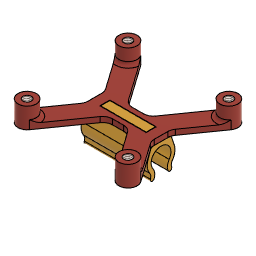
PixRacer Mount v3 (Autodesk Fusion 360 design; units mm, degrees)
Autodesk Fusion 360 part; units mm, degrees
note: some values were not read from the file. Chosen so that the rebuilt part matches the saved one: which face or edge a step refers to; which pieces of a blend or face edit are solid. Set by a fixed rule: which sketch regions a step uses.
sketch "Sketch1" plane through (0, 0, 0) normal (0, 0, 1) x (1, 0, 0)
  circle A0 centre (15.25, 15.25) radius 2.7625
  line L0 (0, 0) -> (0, 23.0197) construction
  line L1 (10, 3) -> (-10, 3)
  line L2 (-10, 3) -> (-10, -3)
  line L3 (-10, -3) -> (10, -3)
  line L4 (10, -3) -> (10, 3)
  line L5 (10, 3) -> (-10, -3) construction
  line L6 (-10, 3) -> (10, -3) construction
  line L7 (10, 3) -> (17.5084, 13.6591)
  line L8 (12.9916, 16.8409) -> (3.2419, 3)
  line L9 (0, 0) -> (10, 0)
  line L10 (10, -3) -> (17.5084, -13.6591)
  circle A1 centre (15.25, -15.25) radius 2.7625
  line L11 (12.9916, -16.8409) -> (3.2419, -3)
  line L12 (-10, 3) -> (-17.5084, 13.6591)
  circle A2 centre (-15.25, 15.25) radius 2.7625
  line L13 (-12.9916, 16.8409) -> (-3.2419, 3)
  line L14 (-10, -3) -> (-17.5084, -13.6591)
  line L15 (-12.9916, -16.8409) -> (-3.2419, -3)
  circle A3 centre (-15.25, -15.25) radius 2.7625
  line L16 (7, 1.5) -> (-7, 1.5)
  line L17 (-7, 1.5) -> (-7, -1.5)
  line L18 (-7, -1.5) -> (7, -1.5)
  line L19 (7, -1.5) -> (7, 1.5)
  line L20 (7, 1.5) -> (-7, -1.5) construction
  line L21 (-7, 1.5) -> (7, -1.5) construction
  dimension "d3" = 5.525
  dimension "d4" = 15.25
  dimension "d5" = 15.25
  dimension "d6" = 20
  dimension "d7" = 6
  dimension "d32" = 3
  dimension "d33" = 3
  constraint coincident L0.start L9.start
  constraint vertical L0
  constraint horizontal L1
  constraint perpendicular L1 L2
  constraint parallel L1 L3
  constraint parallel L2 L4
  constraint coincident L5 L0.start
  constraint coincident L6 L0.start
  constraint coincident A0 L7.end
  constraint tangent A0 L7
  constraint coincident A0 L8.start
  constraint coincident L1 L8.end
  constraint parallel L7 L8
  constraint tangent A0 L8
  constraint midpoint L4 L9.end
  constraint symmetric A0 L9 A1
  constraint symmetric L1.start L9 L3.end
  constraint symmetric L7.end L9 L10.end
  constraint symmetric L8.start L9 L11.start
  constraint symmetric L8.end L9 L11.end
  constraint symmetric A0 L0 A2
  constraint symmetric L0 L1.start L1.end
  constraint symmetric L0 L7.end L12.end
  constraint symmetric L0 L8.start L13.start
  constraint symmetric L0 L8.end L13.end
  constraint symmetric L0 L3.end L2.end
  constraint symmetric L0 L10.end L14.end
  constraint symmetric L0 A1 A3
  constraint symmetric L0 L11.start L15.start
  constraint symmetric L0 L11.end L15.end
  constraint horizontal L16
  constraint perpendicular L16 L17
  constraint parallel L16 L18
  constraint parallel L17 L19
  constraint coincident L20 L0.start
  constraint coincident L21 L0.start
  measures "d3" diameter of A0
  measures "d4" distance of A0.centre L0
  measures "d5" vertical distance of L0.start A0.centre
  measures "d6" distance of L2.end L3.end
  measures "d7" distance of L1.end L2.end
  measures "d32" distance of L16.start L18.end
  measures "d33" distance of L2 L17
extrude "Extrude1" add sketch "Sketch1" along normal blind 1.6 makes body 1
extrude "Extrude2" add sketch "Sketch1" along normal blind 4.6 from surface at 1.6 contours A0 | A2 | A1 | A3 bodies 1
sketch "Sketch2" plane through (0, 0, 6.2) normal (0, 0, 1) x (-1, 0, 0)
  circle A0 centre (15.25, -15.25) radius 2.7625
  point P0 (15.25, -15.25)
  point P1 (-15.25, -15.25)
  point P2 (-15.25, 15.25)
  point P3 (15.25, 15.25)
hole "Hole1" at (-15.25, 15.25, 6.2) at (15.25, 15.25, 6.2) at (15.25, -15.25, 6.2) at (-15.25, -15.25, 6.2) direction (0, 0, -1) diameter 2.529 depth 5 tip angle 180 bodies 1
thread "Thread1" "ISO Metric profile 3.0 M3x0.5 6H"
sketch "Sketch3" plane through (10, 0, 0) normal (1, 0, 0) x (0, 1, 0)
  line L0 (-3, 0) -> (3, 0)
  line L1 (3, 0) -> (3, 1.6)
  line L2 (3, 1.6) -> (-3, 1.6)
  line L3 (-3, 1.6) -> (-3, 0)
  line L4 (0, 0) -> (0, -5.6147) construction
  line L5 (0, -4.2) -> (-3, -4.2) construction
  arc A0 (2.4575, -5.9207) -> (-2.4575, -5.9207) centre (0, -4.2) ccw
  line L6 (-2.4575, -5.9207) -> (0, -4.2) construction
  arc A1 (-2.4575, -9.3622) -> (-2.4575, -5.9207) centre (-4.9149, -7.6415) ccw
  arc A2 (2.4575, -5.9207) -> (2.4575, -9.3622) centre (4.9149, -7.6415) ccw
  arc A3 (-3.4404, -8.6739) -> (-3.4404, -6.609) centre (-4.9149, -7.6415) ccw
  arc A4 (3.4404, -6.609) -> (3.4404, -8.6739) centre (4.9149, -7.6415) ccw
  line L7 (-2.4575, -9.3622) -> (-3.4404, -8.6739)
  line L8 (2.4575, -9.3622) -> (3.4404, -8.6739)
  arc A5 (-1.9743, -8.2356) -> (-2.4575, -5.9207) centre (-4.9149, -7.6415) ccw
  arc A6 (3.4404, -6.609) -> (-3.4404, -6.609) centre (0, -4.2) ccw
  arc A7 (2.4575, -5.9207) -> (1.9743, -8.2356) centre (4.9149, -7.6415) ccw
  line L9 (-3, 0) -> (3, 0)
  line L10 (-1.5, 0) -> (1.5, 0)
  line L11 (3, 0) -> (3.973, -2.8378)
  line L12 (-3, 0) -> (-3.973, -2.8378)
  point P0 (3, 0)
  dimension "d16" = 35
  dimension "d17" = 3
  dimension "d18" = 3
  dimension "d34" = -1.2
  constraint coincident L4.start origin
  constraint perpendicular L0 L4
  constraint coincident L4 L5.start
  constraint perpendicular L4 L5
  constraint coincident L5.start A0.centre
  constraint coincident L5.end A0
  constraint symmetric L4 A0.start A0.end
  constraint tangent A0 A1
  constraint vertical A0.end A1.start
  constraint symmetric L4 A0.end A0.start
  constraint symmetric L4 A1.start A2.end
  constraint symmetric L4 A1 A2
  constraint concentric A1 A3
  constraint concentric A2 A4
  constraint coincident P0 L0.end
  constraint coincident A6 L11.end
  constraint tangent A6 L11
  constraint coincident L0.start L3.end
  constraint coincident A6 L12.end
  constraint tangent A6 L12
  constraint coincident L4.start A6
  measures "d16" angle of L5 L6
  measures "d17" distance of L5.start L5.end
  measures "d18" radius of A1
fillet "Fillet4" radius 1 4 edges at (-13.6591, -12.9916, 1.6) (13.6591, -12.9916, 1.6) (13.6591, 12.9916, 1.6) (-13.6591, 12.9916, 1.6) on bodies 1
fillet "Fillet5" radius 3 8 edges at (10, -3, 0.8) (10, 3, 0.8) (-3.2419, -3, 0.8) (3.2419, -3, 0.8) (-10, 3, 0.8) (-10, -3, 0.8) (3.2419, 3, 0.8) (-3.2419, 3, 0.8) on bodies 1
extrude "Extrude1'" add sketch "Sketch3" against normal up to surface (20 mm away) separate body contours L0 A6 L9 L10 L12 | A0 A1 A2 A3 A4 L7 L8 A5 A6 A7 | L0 A6 L9 L10 L11 makes body 2 in component "Component"
sketch "Sketch1 (2)" plane through (0, 0, 0) normal (0, 0, 1) x (1, 0, 0) in component "Component"
  line L0 (-7, -1.5) -> (-7, 1.5) construction
  line L1 (-7, 1.5) -> (7, 1.5) construction
  line L2 (7, -1.5) -> (-7, -1.5) construction
  line L3 (7, 1.5) -> (7, -1.5) construction
  line L4 (6.9, -1.4) -> (-6.9, -1.4)
  line L5 (-6.9, -1.4) -> (-6.9, 1.4)
  line L6 (-6.9, 1.4) -> (6.9, 1.4)
  line L7 (6.9, 1.4) -> (6.9, -1.4)
  dimension "d37" = 0.1
extrude "Extrude2'" add sketch "Sketch1 (2)" along normal up to surface (1.6 mm away) bodies 2 in component "Component"
fillet "Fillet1" radius 0.6 2 edges at (0, -3.4404, -8.6739) (0, -2.4575, -9.3622) on bodies 2 in component "Component"
fillet "Fillet1" radius 0.6 2 edges at (0, 3.4404, -8.6739) (0, 2.4575, -9.3622) on bodies 2 in component "Component"
fillet "Fillet1" radius 1.0324 2 edges at (0, 3.4404, -8.6739) (0, 3.4404, -6.609) on bodies 2 in component "Component"
component "Component" placed x (1, 0, 0) y (0, 1, 0) z (0, 0, 1) at (0, 0, 0)
equation "d3 = ( 2.7625 * 2 ) * 1 mm"
equation "d4 = ( 30.5 / 2 ) * 1 mm"
equation "d5 = d4"
equation "d18 = d17"
